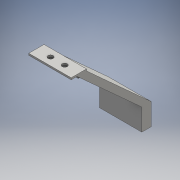
# Autodesk Inventor part: leverArm
Saved by Autodesk Inventor 2016 (Build 200138000, 138)
## iProperties
Created: 2016-05-03
Part Number: leverArm
Material: Generic
Document SubType Name: Modeling
Designer: mkepler
Density: 1 g/cm^3
Appearance: Default
Author: mkepler
Autodesk Inventor part; units mm, degrees
ref_plane "YZ Plane" through (0, 0, 0) normal (1, 0, 0) x (0, 1, 0)
ref_plane "XZ Plane" through (0, 0, 0) normal (0, 1, 0) x (-1, 0, 0)
ref_plane "XY Plane" through (0, 0, 0) normal (0, 0, 1) x (1, 0, 0)
sketch "Sketch1" plane through (0, 0, 0) normal (1, 0, 0) x (0, 1, 0)
  line L0 (0, 0) -> (13, 0)
  line L1 (13, 0) -> (13, -1.5)
  line L2 (13, -1.5) -> (13, -51.5)
  line L3 (13, -51.5) -> (60, -51.5)
  line L4 (13, -1.5) -> (68, -51.5)
  line L5 (68, -51.5) -> (68, -70)
  line L6 (68, -70) -> (60, -70)
  line L7 (60, -70) -> (60, -51.5)
  line L8 (0, 0) -> (0, -1.5)
  line L9 (0, -1.5) -> (5, -1.5)
  line L10 (5, -1.5) -> (60, -51.5)
  dimension "d4" = 13
  dimension "d5" = 1.5
  dimension "d6" = 50
  dimension "d7" = 55
  dimension "d8" = 18.5
  dimension "d9" = 8
  dimension "d10" = 1.5
  dimension "d11" = 5
  constraints: 22 end point, 4 perpendicular, 2 horizontal, 2 vertical, 1 parallel
  measures "d4" distance of L0.start L0.end
  measures "d5" distance of L0.end L1.end
  measures "d6" distance of L1.end L2.end
  measures "d7" distance of L2.end L4.end
  measures "d8" distance of L4.end L5.end
  measures "d9" distance of L5.end L6.end
  measures "d10" distance of L0.start L8.end
  measures "d11" distance of L8.end L9.end
extrude "Extrusion1" add sketch "Sketch1" along normal blind 36 contours L0 L1 L2 L10 L9 L8 | L4 L5 L6 L7 L10 L2
sketch "Sketch3" plane through (0, 60, -70) normal (0, 0, -1) x (-1, 0, 0)
  line L0 (0, 0) -> (-36, 0) projected
  line L1 (-36, 0) -> (-36, 4)
  line L2 (-36, 8) -> (-36, -47) projected
  line L3 (-36, 4) -> (0, 4)
  line L4 (0, 8) -> (0, -47) projected
  line L5 (-8, 7) -> (-28, 7) projected
  line L6 (-18, 7) -> (-18, 0)
  circle A0 centre (-24, 4) radius 2.175
  circle A1 centre (-12, 4) radius 2.175
  point P0 (0, -60)
  dimension "d20" = 4
  dimension "d21" = 4.35
  dimension "d22" = 4.35
  dimension "d23" = 6
  dimension "d24" = 6
  constraints: 6 end point, 4 point on line, 2 centre point, 2 midpoint, 1 perpendicular
  measures "d20" distance of L0.end L1.end
  measures "d21" diameter of A0
  measures "d22" diameter of A1
  measures "d23" distance from line of L6 A0.centre
  measures "d24" distance from line of L6 A1.centre
hole "Hole1" at (24, 64, -70) at (12, 64, -70) direction (0, 0, 1) diameter 4.35 depth 8 tip angle 118
sketch "Sketch5" plane through (0, 0, 0) normal (0, 0, 1) x (1, 0, 0)
  line L0 (0, 0) -> (0, 13)
  line L1 (0, 5) -> (0, 60) projected
  line L2 (0, 13) -> (36, 13) projected
  line L3 (0, 13) -> (36, 13)
  line L4 (36, 5) -> (36, 60) projected
  line L5 (18, 13) -> (18, 0)
  line L6 (0, 0) -> (36, 0) projected
  line L7 (0, 6.5) -> (36, 6.5)
  circle A0 centre (24, 6.5) radius 2.175
  circle A1 centre (12, 6.5) radius 2.175
  dimension "d35" = 13
  dimension "d36" = 4.35
  dimension "d37" = 6
  dimension "d38" = 4.35
  dimension "d39" = 6
  constraints: 8 end point, 5 point on line, 2 centre point, 2 midpoint, 2 perpendicular
  measures "d35" distance of L0.start L0.end
  measures "d36" diameter of A0
  measures "d37" distance from line of L5 A0.centre
  measures "d38" diameter of A1
  measures "d39" distance from line of L5 A1.centre
hole "Hole2" at (24, 6.5, 0) at (12, 6.5, 0) direction (0, 0, -1) diameter 4.35 end through all
sketch "Sketch6" plane through (0, 0, -1.5) normal (0, -1, 0) x (1, 0, 0)
  line L0 (0, 0) -> (6, 0)
  line L1 (0, 0) -> (10.425, 0) projected
  line L2 (25.575, 0) -> (36, 0) projected
  line L3 (36, 0) -> (30, 0)
  line L4 (30, 0) -> (30, -8)
  line L5 (30, -8) -> (6, -8)
  line L6 (6, -8) -> (6, 0)
  line L7 (6, 0) -> (30, 0)
  point P0 (0, 1.5)
  dimension "d47" = 6
  dimension "d48" = 6
  dimension "d49" = 8
  dimension "d50" = 24
  dimension "d51" = 90
  constraints: 12 end point, 2 perpendicular, 2 point on line, 1 collinear
  measures "d47" distance of L0.start L0.end
  measures "d48" distance of L2.end L3.end
  measures "d49" distance of L3.end L4.end
  measures "d50" distance of L4.end L5.end
  measures "d51" angle of L4 L5
extrude "Extrusion3" add sketch "Sketch6" against normal through all
sketch "Sketch7" plane through (0, 0, -1.5) normal (0, -1, 0) x (1, 0, 0)
  line L0 (6, -8) -> (6, 0) projected
  line L1 (30, -8) -> (6, -8) projected
  line L2 (6, 0) -> (30, 0)
  line L3 (30, 0) -> (30, -8)
  line L4 (30, -8) -> (6, -8)
  line L5 (6, -8) -> (6, 0)
  point P0 (0, 1.5)
  dimension "d54" = 24
  constraints: 8 end point, 2 parallel, 1 horizontal, 1 perpendicular
  measures "d54" distance of L1.start L4.end
extrude "Extrusion4" cut sketch "Sketch7" against normal blind 12
body "Solid1"
